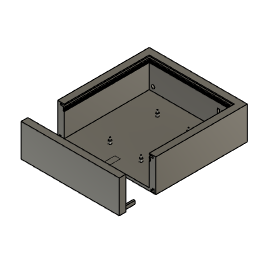
Box v41 (Autodesk Fusion 360 design; units mm, degrees)
Autodesk Fusion 360 part; units mm, degrees
sketch "Box" plane through (0, 0, 0) normal (0, 0, 1) x (1, 0, 0) in component "Box"
  line L0 (90, -90) -> (-90, -90)
  line L1 (-90, -90) -> (-90, 90)
  line L2 (-90, 90) -> (90, 90)
  line L3 (90, 90) -> (90, -90)
  line L4 (90, -90) -> (-90, 90) construction
  line L5 (-90, -90) -> (90, 90) construction
  dimension "d1" = 180
  dimension "d2" = 180
  constraint horizontal L0
  constraint perpendicular L0 L1
  constraint parallel L0 L2
  constraint parallel L1 L3
  constraint coincident L4 origin
  constraint coincident L5 origin
  measures "d1" distance of L1.end L2.end
  measures "d2" distance of L0.end L1.end
extrude "Extrude1" add sketch "Box" along normal blind 60 makes body 1 in component "Box"
sketch "Main Hole" plane through (0, 0, 60) normal (0, 0, 1) x (-1, 0, 0) in component "Box"
  line L0 (-90, -90) -> (90, -90)
  line L1 (90, -90) -> (90, 90)
  line L2 (90, 90) -> (-90, 90)
  line L3 (-90, 90) -> (-90, -90)
  line L4 (-78, 78) -> (78, 78)
  line L5 (78, 78) -> (78, -78)
  line L6 (78, -78) -> (-78, -78)
  line L7 (-78, -78) -> (-78, 78)
  line L8 (-78, 78) -> (78, -78) construction
  line L9 (78, 78) -> (-78, -78) construction
  dimension "d5" = 156
  dimension "d6" = 156
  constraint horizontal L4
  constraint perpendicular L4 L5
  constraint parallel L4 L6
  constraint parallel L5 L7
  constraint coincident L8 origin
  constraint coincident L9 origin
  measures "d5" distance of L5.end L6.end
  measures "d6" distance of L4.end L5.end
extrude "Extrude2" cut sketch "Main Hole" against normal up to surface (55 mm away) contours L4 L5 L6 L7 bodies 1 in component "Box"
sketch "Diffuser Layer" plane through (0, 0, 60) normal (0, 0, 1) x (-1, 0, 0) in component "Box"
  line L0 (-78, -78) -> (-78, 78)
  line L1 (-78, 78) -> (78, 78)
  line L2 (78, 78) -> (78, -78)
  line L3 (78, -78) -> (-78, -78)
  line L4 (-90, -90) -> (90, -90)
  line L5 (90, -90) -> (90, 90)
  line L6 (90, 90) -> (-90, 90)
  line L7 (-90, 90) -> (-90, -90)
  line L8 (-78, 79.9312) -> (78, 79.9312)
  line L9 (78, 79.9312) -> (78, -79.9312)
  line L10 (78, -79.9312) -> (-78, -79.9312)
  line L11 (-78, -79.9312) -> (-78, 79.9312)
  line L12 (-78, 79.9312) -> (78, -79.9312) construction
  line L13 (78, 79.9312) -> (-78, -79.9312) construction
  line L14 (-85, 85) -> (85, 85)
  line L15 (85, 85) -> (85, -85)
  line L16 (85, -85) -> (-85, -85)
  line L17 (-85, -85) -> (-85, 85)
  line L18 (-85, 85) -> (85, -85) construction
  line L19 (85, 85) -> (-85, -85) construction
  dimension "d9" = 170
  dimension "d10" = 170
  constraint horizontal L8
  constraint perpendicular L8 L9
  constraint parallel L8 L10
  constraint parallel L9 L11
  constraint coincident L0 L8.start
  constraint coincident L12 origin
  constraint coincident L13 origin
  constraint horizontal L14
  constraint perpendicular L14 L15
  constraint parallel L14 L16
  constraint parallel L15 L17
  constraint coincident L18 origin
  constraint coincident L19 origin
  measures "d9" distance of L15.end L16.end
  measures "d10" distance of L14.end L15.end
extrude "Extrude3" cut sketch "Diffuser Layer" against normal blind 3 from surface at -2 contours L0 L1 L2 L3 L9 L11 | L3 L9 L10 L11 | L1 L8 L9 L11 | L14 L15 L16 L17 bodies 1 in component "Box"
sketch "Matrix Top Layer" plane through (0, 0, 60) normal (0, 0, 1) x (-1, 0, 0) in component "Box"
  line L0 (-78, -78) -> (-78, 78)
  line L1 (-78, 78) -> (78, 78)
  line L2 (78, 78) -> (78, -78)
  line L3 (78, -78) -> (-78, -78)
  line L4 (-90, -90) -> (90, -90)
  line L5 (90, -90) -> (90, 90)
  line L6 (90, 90) -> (-90, 90)
  line L7 (-90, 90) -> (-90, -90)
  line L8 (80, -80) -> (-80, -80)
  line L9 (-80, -80) -> (-80, 80)
  line L10 (-80, 80) -> (80, 80)
  line L11 (80, 80) -> (80, -80)
  line L12 (80, -80) -> (-80, 80) construction
  line L13 (-80, -80) -> (80, 80) construction
  dimension "d14" = 160
  dimension "d15" = 160
  constraint horizontal L8
  constraint perpendicular L8 L9
  constraint parallel L8 L10
  constraint parallel L9 L11
  constraint coincident L12 origin
  constraint coincident L13 origin
  measures "d14" distance of L9.end L10.end
  measures "d15" distance of L8.end L9.end
extrude "Extrude4" cut sketch "Matrix Top Layer" against normal blind 1 from surface at -7 contours L0 L1 L2 L3 | L8 L9 L10 L11 bodies 1 in component "Box"
sketch "Matrix Top Layer (2)" plane through (0, 0, 52) normal (0, 0, 1) x (-1, 0, 0)
  line L0 (78, 78) -> (78, -78)
  line L1 (78, -78) -> (-78, -78)
  line L2 (-78, -78) -> (-78, 78)
  line L3 (-78, 78) -> (78, 78)
  line L4 (80, 80) -> (-80, 80)
  line L5 (-80, 80) -> (-80, -80)
  line L6 (-80, -80) -> (80, -80)
  line L7 (80, -80) -> (80, 80)
extrude "Extrude5" cut sketch "Matrix Top Layer (2)" against normal blind 1 from surface at -1 bodies 1 in component "Box"
sketch "Matrix Bottom Layer" plane through (0, 0, 50) normal (0, 0, 1) x (-1, 0, 0)
  line L0 (-78, -78) -> (-78, 78)
  line L1 (-78, 78) -> (78, 78)
  line L2 (78, 78) -> (78, -78)
  line L3 (78, -78) -> (-78, -78)
  line L4 (80, -80) -> (80, 80)
  line L5 (80, 80) -> (-80, 80)
  line L6 (-80, 80) -> (-80, -80)
  line L7 (-80, -80) -> (80, -80)
  line L8 (80, -80) -> (-80, -80)
  line L9 (-80, -80) -> (-80, 80)
  line L10 (-80, 80) -> (80, 80)
  line L11 (80, 80) -> (80, -80)
  constraint horizontal L8
  constraint vertical L9
  constraint horizontal L10
  constraint vertical L11
  constraint coincident L5.end L6.start
  constraint coincident L4.start L7.end
extrude "Extrude11" cut sketch "Matrix Bottom Layer" against normal blind 1 from surface at -1 contours L0 L1 L2 L3 | L4 L5 L6 L7 L8 L9 L10 L11 bodies 1 in component "Box"
sketch "Cable Hole" plane through (0, 90, 0) normal (0, 1, 0) x (-1, 0, 0)
  line L0 (-90, 0) -> (90, 0)
  line L1 (90, 0) -> (90, 60)
  line L2 (90, 60) -> (-90, 60)
  line L3 (-90, 60) -> (-90, 0)
  circle A0 centre (71, 13) radius 3
  dimension "d23" = 6
  measures "d23" diameter of A0
extrude "Extrude6" cut sketch "Cable Hole" against normal blind 12 contours A0 bodies 1 in component "Box"
ref_plane "WorkPlane1" through (0, -78, 30) normal (0, -1, 0) x (1, 0, 0)
split "Split1" by plane through (0, -78, 30) normal (0, -1, 0) bodies 1 makes body 2 at (30, -90, 40) in component "Box"
move_body "Move1" bodies 2 to x (1, 0, 0) y (0, 1, 0) z (0, 0, 1) at (0, -35, 0) in component "Box"
move_body "Move2" bodies 2 to x (1, 0, 0) y (0, 1, 0) z (0, 0, 1) at (0, -130, 0) in component "Box"
sketch "Inlets" plane through (0, -78, 25) normal (0, -1, 0) x (1, 0, 0)
  line L0 (87, -24) -> (84, -24)
  line L1 (84, -24) -> (84, -18)
  line L2 (84, -18) -> (87, -18)
  line L3 (87, -18) -> (87, -24)
  line L4 (87, -24) -> (81, -24)
  line L5 (81, -24) -> (81, -21)
  line L6 (81, -21) -> (87, -21)
  line L7 (87, -21) -> (87, -24)
  line L8 (-87, -24) -> (-84, -24)
  line L9 (-84, -24) -> (-84, -18)
  line L10 (-84, -18) -> (-87, -18)
  line L11 (-87, -18) -> (-87, -24)
  line L12 (-87, -24) -> (-81, -24)
  line L13 (-81, -24) -> (-81, -21)
  line L14 (-81, -21) -> (-87, -21)
  line L15 (-87, -21) -> (-87, -24)
  line L16 (-5, -21) -> (5, -21)
  line L17 (5, -21) -> (5, -24)
  line L18 (5, -24) -> (-5, -24)
  line L19 (-5, -24) -> (-5, -21)
  dimension "d52" = 3
  dimension "d53" = 6
  dimension "d54" = 6
  dimension "d55" = 3
  dimension "d56" = 3
  dimension "d57" = 6
  dimension "d58" = 6
  dimension "d59" = 3
  constraint horizontal L0
  constraint vertical L1
  constraint horizontal L2
  constraint vertical L3
  constraint horizontal L4
  constraint vertical L5
  constraint horizontal L6
  constraint vertical L7
  constraint horizontal L8
  constraint vertical L9
  constraint horizontal L10
  constraint vertical L11
  constraint horizontal L12
  constraint vertical L13
  constraint horizontal L14
  constraint vertical L15
  constraint horizontal L16
  constraint vertical L17
  constraint horizontal L18
  constraint vertical L19
  measures "d52" distance of L0.start L0.end
  measures "d53" distance of L0.start L2.end
  measures "d54" distance of L0.start L4.end
  measures "d55" distance of L0.start L6.end
  measures "d56" distance of L8.start L8.end
  measures "d57" distance of L8.start L10.end
  measures "d58" distance of L8.start L12.end
  measures "d59" distance of L8.start L14.end
extrude "Extrude9" cut sketch "Inlets" against normal blind 20 bodies 1 in component "Box"
sketch "Studs" plane through (0, -243, 0) normal (0, 1, 0) x (-1, 0, 0)
  line L0 (90, 60) -> (-90, 60)
  line L1 (-90, 60) -> (-90, 0)
  line L2 (-90, 0) -> (90, 0)
  line L3 (90, 0) -> (90, 60)
  line L4 (-85, 58) -> (85, 58)
  line L5 (85, 58) -> (85, 55)
  line L6 (85, 55) -> (-85, 55)
  line L7 (-85, 55) -> (-85, 58)
  line L8 (-80, 53) -> (80, 53)
  line L9 (80, 53) -> (80, 52)
  line L10 (80, 52) -> (-80, 52)
  line L11 (-80, 52) -> (-80, 53)
  line L12 (-80, 51) -> (80, 51)
  line L13 (80, 51) -> (80, 50)
  line L14 (80, 50) -> (-80, 50)
  line L15 (-80, 50) -> (-80, 51)
  line L16 (-84, 1) -> (-84, 7)
  line L17 (-81, 4) -> (-87, 4)
  line L18 (-87, 7) -> (-87, 1)
  line L19 (-87, 4) -> (-87, 1)
  line L20 (87, 1) -> (84, 1)
  line L21 (-87, 1) -> (-84, 1)
  line L22 (87, 7) -> (87, 1)
  line L23 (81, 4) -> (87, 4)
  line L24 (-5, 1) -> (-5, 4)
  line L25 (-5, 4) -> (5, 4)
  line L26 (87, 1) -> (81, 1)
  line L27 (-81, 1) -> (-81, 4)
  line L28 (81, 1) -> (81, 4)
  line L29 (5, 1) -> (-5, 1)
  line L30 (84, 7) -> (87, 7)
  line L31 (5, 4) -> (5, 1)
  line L32 (87, 4) -> (87, 1)
  line L33 (84, 1) -> (84, 7)
  line L34 (-87, 1) -> (-81, 1)
  line L35 (-84, 7) -> (-87, 7)
  line L36 (-80, 49) -> (80, 49)
  line L37 (80, 49) -> (80, 48)
  line L38 (80, 48) -> (-80, 48)
  line L39 (-80, 48) -> (-80, 49)
  point P0 (0, 25)
  dimension "d64" = 3
  dimension "d65" = 6
  dimension "d66" = 6
  dimension "d67" = 3
  dimension "d68" = 3
  dimension "d69" = 6
  dimension "d70" = 6
  dimension "d71" = 3
  constraint horizontal L20
  constraint vertical L33
  constraint horizontal L30
  constraint vertical L22
  constraint horizontal L26
  constraint vertical L28
  constraint horizontal L23
  constraint vertical L32
  constraint horizontal L21
  constraint vertical L16
  constraint horizontal L35
  constraint vertical L18
  constraint horizontal L34
  constraint vertical L27
  constraint horizontal L17
  constraint vertical L19
  constraint horizontal L25
  constraint vertical L31
  constraint horizontal L29
  constraint vertical L24
  measures "d64" distance of L20.end L20.start
  measures "d65" distance of L22.start L20.start
  measures "d66" distance of L20.start L26.end
  measures "d67" distance of L20.start L23.end
  measures "d68" distance of L18.end L16.start
  measures "d69" distance of L18.end L18.start
  measures "d70" distance of L18.end L27.start
  measures "d71" distance of L18.end L17.end
extrude "Extrude10" add sketch "Studs" along normal blind 20 contours L16 L17 L18 L19 L21 L34 | L16 L17 L27 L34 | L16 L17 L18 L35 | L20 L22 L23 L26 L32 L33 | L23 L26 L28 L33 | L22 L23 L30 L33 | L24 L25 L29 L31 bodies 2 in component "Box"
move_body "Move4" bodies 2 to x (1, 0, 0) y (0, 1, 0) z (0, 0, 1) at (0, 110, 0) in component "Box"
sketch "Ventilation" plane through (0, 90, 0) normal (0, 1, 0) x (-1, 0, 0)
  circle A0 centre (71, 13) radius 3
  line L0 (-90, 0) -> (90, 0)
  line L1 (90, 0) -> (90, 60)
  line L2 (90, 60) -> (-90, 60)
  line L3 (-90, 60) -> (-90, 0)
  line L4 (-75, 8) -> (-71, 8)
  line L5 (-71, 8) -> (-71, 38)
  line L6 (-71, 38) -> (-75, 38)
  line L7 (-75, 38) -> (-75, 8)
  line L8 (-67, 8) -> (-63, 8)
  line L9 (-63, 8) -> (-63, 38)
  line L10 (-63, 38) -> (-67, 38)
  line L11 (-67, 38) -> (-67, 8)
  line L12 (-59, 8) -> (-55, 8)
  line L13 (-55, 8) -> (-55, 38)
  line L14 (-55, 38) -> (-59, 38)
  line L15 (-59, 38) -> (-59, 8)
  line L16 (-51, 8) -> (-47, 8)
  line L17 (-47, 8) -> (-47, 38)
  line L18 (-47, 38) -> (-51, 38)
  line L19 (-51, 38) -> (-51, 8)
  dimension "d83" = 4
  dimension "d84" = 30
  dimension "d85" = 4
  dimension "d86" = 30
  dimension "d87" = 4
  dimension "d88" = 30
  dimension "d89" = 4
  dimension "d90" = 30
  constraint horizontal L4
  constraint vertical L5
  constraint horizontal L6
  constraint vertical L7
  constraint horizontal L8
  constraint vertical L9
  constraint horizontal L10
  constraint vertical L11
  constraint horizontal L12
  constraint vertical L13
  constraint horizontal L14
  constraint vertical L15
  constraint horizontal L16
  constraint vertical L17
  constraint horizontal L18
  constraint vertical L19
  measures "d83" distance of L4.start L4.end
  measures "d84" distance of L4.start L6.end
  measures "d85" distance of L8.start L8.end
  measures "d86" distance of L8.start L10.end
  measures "d87" distance of L12.start L12.end
  measures "d88" distance of L12.start L14.end
  measures "d89" distance of L16.start L16.end
  measures "d90" distance of L16.start L18.end
extrude "Extrude12" cut sketch "Ventilation" against normal up to surface (12 mm away) contours L4 L5 L6 L7 | L8 L9 L10 L11 | L12 L13 L14 L15 | L16 L17 L18 L19 bodies 1 in component "Box"
sketch "Board" plane through (0, 0, 5) normal (0, 0, 1) x (-1, 0, 0)
  line L0 (78, -78) -> (78, 78)
  line L1 (78, 78) -> (-78, 78)
  line L2 (-78, 78) -> (-78, -78)
  line L3 (-78, -78) -> (78, -78)
  line L4 (32, 47) -> (-32, 47)
  line L5 (-32, 47) -> (-32, -47)
  line L6 (-32, -47) -> (32, -47)
  line L7 (32, -47) -> (32, 47)
  line L8 (32, 47) -> (-32, -47) construction
  line L9 (-32, 47) -> (32, -47) construction
  circle A0 centre (28.5, -43.5) radius 1
  circle A1 centre (28.5, -43.5) radius 2.5
  circle A2 centre (-28.5, -43.5) radius 500
  circle A3 centre (-28.5, -43.5) radius 1
  circle A4 centre (-28.5, -43.5) radius 2.5
  circle A5 centre (-28.5, 43.5) radius 1
  circle A6 centre (-28.5, 43.5) radius 2.5
  circle A7 centre (28.5, 43.5) radius 1
  circle A8 centre (28.5, 43.5) radius 2.5
  dimension "d93" = 64
  dimension "d94" = 94
  dimension "d123" = 2
  dimension "d124" = 5
  dimension "d126" = 2
  dimension "d127" = 5
  dimension "d128" = 2
  dimension "d129" = 5
  dimension "d130" = 2
  dimension "d131" = 5
  constraint horizontal L4
  constraint perpendicular L4 L5
  constraint parallel L4 L6
  constraint parallel L5 L7
  constraint coincident L8 origin
  constraint coincident L9 origin
  constraint concentric A0 A1
  constraint concentric A2 A3
  constraint concentric A3 A4
  constraint concentric A5 A6
  constraint concentric A7 A8
  measures "d93" distance of L5.end L6.end
  measures "d94" distance of L4.end L5.end
  measures "d123" diameter of A0
  measures "d124" diameter of A1
  measures "d126" diameter of A3
  measures "d127" diameter of A4
  measures "d128" diameter of A5
  measures "d129" diameter of A6
  measures "d130" diameter of A7
  measures "d131" diameter of A8
extrude "Extrude14" add sketch "Board" along normal blind 10 contours A0 | A3 | A5 | A7 bodies 1 in component "Box"
extrude "Extrude13" add sketch "Board" along normal blind 5 contours A1 | A4 | A6 | A8 bodies 1 in component "Box"
cylinder "CylinderPrimitive1" add diameter 5 height 4 placed x (1, 0, 0) y (0, 1, 0) z (0, 0, 1) at (-105, -100, 5) separate body makes body 3
sketch "Cap Extrude" plane through (0, 0, 9) normal (0, 0, 1) x (-1, 0, 0)
  circle A0 centre (105, 100) radius 2.5
  circle A1 centre (105, 100) radius 1
  dimension "d112" = 2
  constraint concentric A0 A1
  measures "d112" diameter of A1
extrude "Extrude2'" cut sketch "Cap Extrude" against normal blind 3 contours A1 bodies 3
copy_body "CopyPasteBodies1" bodies 3 makes body 4
move_body "Move1'" bodies 4 to x (1, 0, 0) y (0, 1, 0) z (0, 0, 1) at (-5.5, 0, 0)
copy_body "CopyPasteBodies2" bodies 4 3 makes body 5 makes body 6
move_body "Move2'" bodies 6 5 to x (1, 0, 0) y (0, 1, 0) z (0, 0, 1) at (0, -5.5, 0)
move_body "Move3" bodies 3 4 5 6 to x (1, 0, 0) y (0, 1, 0) z (0, 0, 1) at (0, 0, -5)
component "Box" placed x (1, 0, 0) y (0, 1, 0) z (0, 0, 1) at (0, 0, 0)
equation "d5 = 160 mm - 2 * 2 mm"
equation "d6 = 16 cm - 2 * 2 mm"
equation "d16 = 0 mm - 2 mm - 3 mm - 2 mm"
equation "doveTailAngle = 90 deg + DoveTailAngle"
equation "DoveTailAngle = 10 deg"
named bodies: "Main", "Opener", "Holder Cap 1", "Holder Cap", "Holder Cap 2", "Holder Cap (1)", "Holder Cap (2)", "Holder Cap 3", "Holder Cap 4"
